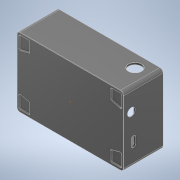
# Autodesk Inventor part: enclosure_bot
Saved by Autodesk Inventor 2021 (Build 250183000, 183)
## iProperties
Created: 2020-12-16
Part Number: enclosure_bot
Material: Generic
Document SubType Name: Modeling
Designer: oskar
Density: 1 g/cm^3
Appearance: Default
Author: oskar
## iProperties of the stored document _3DPrint.ipt
Created: 2020-12-16
Part Number: _3DPrint
Material: Generic
Document SubType Name: Modeling
Designer: oskar
Density: 1 g/cm^3
Appearance: Default
Author: oskar
Autodesk Inventor part; units mm, degrees
ref_plane "YZ Plane" through (0, 0, 0) normal (1, 0, 0) x (0, 1, 0)
ref_plane "XZ Plane" through (0, 0, 0) normal (0, 1, 0) x (-1, 0, 0)
ref_plane "XY Plane" through (0, 0, 0) normal (0, 0, 1) x (1, 0, 0)
ref_plane "Work Plane1" through (-0.485, 4.902, 9.06) normal (0, 0, 1) x (1, 0, 0)
sketch "Sketch1" plane through (-0.485, 4.902, 9.06) normal (0, 0, 1) x (1, 0, 0)
  line L0 (-52.815, 27.598) -> (47.185, 27.598)
  line L1 (47.185, 27.598) -> (47.185, -37.402)
  line L2 (47.185, -37.402) -> (-52.815, -37.402)
  line L3 (-52.815, -37.402) -> (-52.815, 27.598)
  line L4 (-52.815, 27.598) -> (47.185, -37.402) construction
  line L5 (47.185, 27.598) -> (-52.815, -37.402) construction
  line L6 (46.185, -13.982) -> (46.185, -20.322) projected
  line L7 (0.485, -4.902) -> (-19.0054, -4.902) construction
  point P0 (-2.815, -4.902)
  point P1 (-2.815, -4.902)
  dimension "d0" = 100
  dimension "d1" = 65
  dimension "d2" = 1
  constraints: 14 end point, 3 midpoint, 2 horizontal, 2 parallel, 1 perpendicular, 1 point on line
  measures "d0" distance of L0.start L0.end
  measures "d1" distance of L2.end L0.start
  measures "d2" distance between parallel lines of L6 L1
extrude "Extrusion1" add sketch "Sketch1" along normal blind 2
sketch "Sketch2" plane through (-0.485, 4.902, 11.06) normal (0, 0, 1) x (1, 0, 0)
  line L0 (36.185, 25.098) -> (44.185, 25.098)
  line L1 (45.185, 24.098) -> (45.185, 14.0681)
  line L2 (43.9425, 13.098) -> (35.9425, 15.098)
  line L3 (35.185, 16.0681) -> (35.185, 24.098)
  arc A0 (36.185, 25.098) -> (35.185, 24.098) centre (36.185, 24.098) ccw
  arc A1 (45.185, 24.098) -> (44.185, 25.098) centre (44.185, 24.098) ccw
  arc A2 (43.9425, 13.098) -> (45.185, 14.0681) centre (44.185, 14.0681) ccw
  arc A3 (35.185, 16.0681) -> (35.9425, 15.098) centre (36.185, 16.0681) ccw
  line L4 (-2.815, -4.902) -> (-2.815, 4.2729) construction
  line L5 (-2.815, -4.902) -> (-9.8185, -4.902) construction
  line L6 (-41.815, 25.098) -> (-49.815, 25.098)
  line L7 (-50.815, 24.098) -> (-50.815, 14.0681)
  line L8 (-49.5725, 13.098) -> (-41.5725, 15.098)
  line L9 (-40.815, 16.0681) -> (-40.815, 24.098)
  arc A4 (-40.815, 24.098) -> (-41.815, 25.098) centre (-41.815, 24.098) ccw
  arc A5 (-49.815, 25.098) -> (-50.815, 24.098) centre (-49.815, 24.098) ccw
  arc A6 (-50.815, 14.0681) -> (-49.5725, 13.098) centre (-49.815, 14.0681) ccw
  arc A7 (-41.5725, 15.098) -> (-40.815, 16.0681) centre (-41.815, 16.0681) ccw
  line L10 (36.185, -34.902) -> (44.185, -34.902)
  line L11 (45.185, -33.902) -> (45.185, -23.8721)
  line L12 (43.9425, -22.902) -> (35.9425, -24.902)
  line L13 (35.185, -25.8721) -> (35.185, -33.902)
  arc A8 (35.185, -33.902) -> (36.185, -34.902) centre (36.185, -33.902) ccw
  arc A9 (44.185, -34.902) -> (45.185, -33.902) centre (44.185, -33.902) ccw
  arc A10 (45.185, -23.8721) -> (43.9425, -22.902) centre (44.185, -23.8721) ccw
  arc A11 (35.9425, -24.902) -> (35.185, -25.8721) centre (36.185, -25.8721) ccw
  line L14 (-41.815, -34.902) -> (-49.815, -34.902)
  line L15 (-50.815, -33.902) -> (-50.815, -23.8721)
  line L16 (-49.5725, -22.902) -> (-41.5725, -24.902)
  line L17 (-40.815, -25.8721) -> (-40.815, -33.902)
  arc A12 (-41.815, -34.902) -> (-40.815, -33.902) centre (-41.815, -33.902) ccw
  arc A13 (-50.815, -33.902) -> (-49.815, -34.902) centre (-49.815, -33.902) ccw
  arc A14 (-49.5725, -22.902) -> (-50.815, -23.8721) centre (-49.815, -23.8721) ccw
  arc A15 (-40.815, -25.8721) -> (-41.5725, -24.902) centre (-41.815, -25.8721) ccw
  line L18 (47.185, -37.402) -> (47.185, 27.598) projected
  line L19 (-52.815, -37.402) -> (47.185, -37.402) projected
  point P0 (0.485, -4.902)
  dimension "d5" = 1
  dimension "d6" = 10
  dimension "d7" = 10
  dimension "d8" = 12
  dimension "d9" = 60
  dimension "d10" = 96
  dimension "d11" = 2
  dimension "d12" = 2.5
  constraints: 36 end point, 36 symmetric about line, 32 point on circle, 16 centre point, 8 tangent, 3 equal radius, 2 horizontal, 1 parallel, 1 perpendicular, 1 vertical, 12 other
  measures "d5" radius of A0
  measures "d6" distance between parallel lines of L3 L1
  measures "d7" distance from line of L2.end L0
  measures "d8" distance from line of L2.start L0
  measures "d9" distance between parallel lines of L0 L10
  measures "d10" distance between parallel lines of L7 L1
  measures "d11" distance between parallel lines of L18 L11
  measures "d12" distance between parallel lines of L19 L10
extrude "top" cut sketch "Sketch2" against normal blind 1.2
sketch "Sketch4" plane through (46.7, -32.5, 9.06) normal (1, 0, 0) x (0, 0, -1)
  line L0 (5.85, 17.08) -> (5.7, 17.08) construction
  line L1 (5.85, 17.08) -> (5.85, 23.42) construction
  line L2 (5.85, 23.42) -> (5.7, 23.42) construction
  line L3 (5.7, 23.42) -> (5.7, 17.08) construction
  arc A0 (5.7, 17.08) -> (7, 15.78) centre (7, 17.08) ccw construction
  line L4 (7, 15.93) -> (7, 15.78) construction
  arc A1 (5.85, 17.08) -> (7, 15.93) centre (7, 17.08) ccw construction
  line L5 (5.85, 17.08) -> (5.7, 17.08) construction
  line L6 (7.71, 15.93) -> (7.71, 15.78) construction
  line L7 (7.71, 15.93) -> (7, 15.93) construction
  line L8 (7, 15.93) -> (7, 15.78) construction
  line L9 (7, 15.78) -> (7.71, 15.78) construction
  arc A2 (7.71, 15.78) -> (9.01, 17.08) centre (7.71, 17.08) ccw construction
  line L10 (8.86, 17.08) -> (9.01, 17.08) construction
  arc A3 (7.71, 15.93) -> (8.86, 17.08) centre (7.71, 17.08) ccw construction
  line L11 (7.71, 15.93) -> (7.71, 15.78) construction
  line L12 (8.86, 20.6) -> (9.01, 20.6) construction
  line L13 (8.86, 20.6) -> (8.86, 17.08) construction
  line L14 (8.86, 17.08) -> (9.01, 17.08) construction
  line L15 (9.01, 17.08) -> (9.01, 20.6) construction
  arc A4 (7, 24.72) -> (5.7, 23.42) centre (7, 23.42) ccw construction
  line L16 (5.85, 23.42) -> (5.7, 23.42) construction
  arc A5 (7, 24.57) -> (5.85, 23.42) centre (7, 23.42) ccw construction
  line L17 (7, 24.57) -> (7, 24.72) construction
  line L18 (7, 24.57) -> (7, 24.72) construction
  line L19 (7, 24.57) -> (7.71, 24.57) construction
  line L20 (7.71, 24.57) -> (7.71, 24.72) construction
  line L21 (7.71, 24.72) -> (7, 24.72) construction
  arc A6 (9.01, 23.42) -> (7.71, 24.72) centre (7.71, 23.42) ccw construction
  line L22 (7.71, 24.57) -> (7.71, 24.72) construction
  arc A7 (8.86, 23.42) -> (7.71, 24.57) centre (7.71, 23.42) ccw construction
  line L23 (8.86, 23.42) -> (9.01, 23.42) construction
  line L24 (8.86, 23.42) -> (9.01, 23.42) construction
  line L25 (8.86, 23.42) -> (8.86, 20.65) construction
  line L26 (8.86, 20.65) -> (9.01, 20.65) construction
  line L27 (9.01, 20.65) -> (9.01, 23.42) construction
  line L28 (0, 0) -> (0, 65) projected
  line L29 (0, 0) -> (35, 0)
  line L30 (35, 0) -> (35, 65)
  line L31 (35, 65) -> (0, 65)
  line L32 (0, 65) -> (0, 0)
  circle A8 centre (5.3355, 45.2339) radius 1 construction
  circle A9 centre (5.3355, 45.2339) radius 3.5
  line L33 (7.71, 15.58) -> (7, 15.58)
  line L34 (5.5, 17.08) -> (5.5, 23.42)
  line L35 (7, 24.92) -> (7.71, 24.92)
  line L36 (9.21, 23.42) -> (9.21, 17.08)
  line L37 (9.21, 15.58) -> (5.5, 24.92) construction
  line L38 (5.5, 15.58) -> (9.21, 24.92) construction
  arc A10 (5.5, 17.08) -> (7, 15.58) centre (7, 17.08) ccw
  arc A11 (7.71, 15.58) -> (9.21, 17.08) centre (7.71, 17.08) ccw
  arc A12 (7, 24.92) -> (5.5, 23.42) centre (7, 23.42) ccw
  arc A13 (9.21, 23.42) -> (7.71, 24.92) centre (7.71, 23.42) ccw
  line L39 (1.66, 38.1339) -> (9.06, 38.1339)
  line L40 (9.06, 38.1339) -> (9.06, 49.1339)
  line L41 (9.06, 49.1339) -> (1.66, 49.1339)
  line L42 (1.66, 49.1339) -> (1.66, 38.1339)
  line L43 (1.66, 38.1339) -> (9.06, 49.1339) construction
  line L44 (9.06, 38.1339) -> (1.66, 49.1339) construction
  line L45 (8.0855, 38.9489) -> (2.0155, 38.9489) construction
  line L46 (2, 54.598) -> (5.6442, 54.5983) construction
  line L47 (2, 54.598) -> (2, 37.402) construction
  line L48 (9.06, 60) -> (9.06, 5) construction
  line L49 (5.6442, 37.4017) -> (2, 37.402) construction
  point P0 (9.06, 32.5)
  point P1 (7.355, 20.25)
  point P2 (5.36, 43.6339)
  dimension "d15" = 35
  dimension "d16" = 7
  dimension "d17" = 1.5
  dimension "d18" = 0.2
  dimension "d19" = 0.2
  dimension "d20" = 0.2
  dimension "d21" = 0.2
  dimension "d22" = 7.4
  dimension "d23" = 11
  dimension "d24" = 3.9
  constraints: 32 end point, 9 point on line, 8 point on circle, 8 tangent, 6 parallel, 5 centre point, 4 midpoint, 3 equal radius, 3 horizontal, 3 perpendicular, 1 coincident, 1 collinear
  measures "d15" distance of L30.end L31.end
  measures "d16" diameter of A9
  measures "d17" radius of A10
  measures "d18" distance between parallel lines of L21 L35
  measures "d19" distance between parallel lines of L33 L9
  measures "d20" distance between parallel lines of L15 L36
  measures "d21" distance between parallel lines of L34 L3
  measures "d22" distance between parallel lines of L42 L48
  measures "d23" distance between parallel lines of L39 L41
  measures "d24" distance from line of A8.centre L41
extrude "Extrusion3" add sketch "Sketch4" against normal blind 1.6 contours L28 L31 L30 L29
sketch "Sketch6" plane through (46.7, -32.5, 11.06) normal (1, 0, 0) x (0, 0, -1)
  line L0 (3.66, 38.1339) -> (3.66, 49.1339) projected
  line L1 (3.66, 49.1339) -> (11.06, 49.1339) projected
  line L2 (11.06, 49.1339) -> (11.06, 38.1339) projected
  line L3 (11.06, 38.1339) -> (3.66, 38.1339) projected
  line L4 (11.21, 23.42) -> (11.21, 17.08) projected
  arc A0 (9.71, 15.58) -> (11.21, 17.08) centre (9.71, 17.08) ccw projected
  line L5 (9.71, 15.58) -> (9, 15.58) projected
  arc A1 (7.5, 17.08) -> (9, 15.58) centre (9, 17.08) ccw projected
  line L6 (7.5, 17.08) -> (7.5, 23.42) projected
  arc A2 (9, 24.92) -> (7.5, 23.42) centre (9, 23.42) ccw projected
  line L7 (9, 24.92) -> (9.71, 24.92) projected
  arc A3 (11.21, 23.42) -> (9.71, 24.92) centre (9.71, 23.42) ccw projected
  line L8 (37, 65) -> (0, 65) projected
  line L9 (0, 0) -> (0, 65) projected
  line L10 (37, 0) -> (0, 0) projected
  line L11 (37, 0) -> (37, 65) projected
  circle A4 centre (7.3355, 45.2339) radius 1 projected
  circle A5 centre (7.3355, 45.2339) radius 3.5
  point P0 (11.06, 32.5)
  dimension "d27" = 7
  constraints: 1 centre point, 1 coincident
  measures "d27" diameter of A5
extrude "Extrusion4" add sketch "Sketch6" against normal blind 0.4 contours L0 L1 L2 L3
sketch "Sketch7" plane through (-53.3, 32.5, 11.06) normal (0, 1, 0) x (1, 0, 0)
  line L0 (98.4, 37) -> (98.4, 2) projected
  line L1 (98.4, 2) -> (0, 2)
  line L2 (0, 2) -> (0, 37)
  line L3 (0, 37) -> (98.4, 37)
  line L4 (98.4, 37) -> (98.4, 2)
  point P0 (53.3, 11.06)
  constraints: 8 end point, 2 parallel, 1 horizontal, 1 perpendicular
extrude "Extrusion5" add sketch "Sketch7" against normal blind 2
sketch "Sketch8" plane through (-53.3, -32.5, 11.06) normal (0, -1, 0) x (1, 0, 0)
  line L0 (0, -2) -> (98.4, -2)
  line L1 (98.4, -2) -> (98.4, -37)
  line L2 (98.4, -37) -> (0, -37)
  line L3 (0, -37) -> (0, -2)
  point P0 (53.3, -11.06)
  constraints: 8 end point, 2 coincident, 2 parallel, 1 horizontal, 1 perpendicular
extrude "Extrusion6" add sketch "Sketch8" against normal blind 2
sketch "Sketch9" plane through (-53.3, -32.5, 11.06) normal (-1, 0, 0) x (0, 0, 1)
  line L0 (-37, 63) -> (-2, 63)
  line L1 (-2, 63) -> (-2, 2)
  line L2 (-2, 2) -> (-37, 2)
  line L3 (-37, 2) -> (-37, 63)
  point P0 (-11.06, 32.5)
  constraints: 8 end point, 3 coincident, 2 parallel, 1 horizontal, 1 perpendicular
extrude "Extrusion7" add sketch "Sketch9" against normal blind 2
fillet "Fillet1" radius 3 8 edges at (-53.3, 32.5, -7.44) (-53.3, -32.5, -7.44) (46.7, 32.5, -7.44) (-51.3, 30.5, -8.44) (-51.3, -30.5, -8.44) (45.1, -30.5, -8.44) (46.7, -32.5, -7.44) (45.1, 30.5, -8.44)
fillet "Fillet2" radius 0.3 40 edges at (45.8213, 31.6213, 11.06) (-3.3, 32.5, 11.06) (-52.4213, 31.6213, 11.06) (-53.3, 0, 11.06) (-52.4213, -31.6213, 11.06) (-3.3, -32.5, 11.06) (45.8213, -31.6213, 11.06) (46.7, 0, 11.06) (34.9118, 20.3547, 11.06) (34.7, 24.9851, 11.06) (34.9929, 29.7071, 11.06) (39.7, 30, 11.06) (44.4071, 29.7071, 11.06) (44.7, 23.9851, 11.06) (44.3154, 18.1819, 11.06) (39.4575, 19, 11.06) (34.9118, -20.3547, 11.06) (39.4575, -19, 11.06) (44.3154, -18.1819, 11.06) (44.7, -23.9851, 11.06) (44.4071, -29.7071, 11.06) (39.7, -30, 11.06) (34.9929, -29.7071, 11.06) (34.7, -24.9851, 11.06) (-41.5929, -29.7071, 11.06) (-46.3, -30, 11.06) (-51.0071, -29.7071, 11.06) (-51.3, -23.9851, 11.06) (-50.9154, -18.1819, 11.06) (-46.0575, -19, 11.06) (-41.5118, -20.3547, 11.06) (-41.3, -24.9851, 11.06) (-50.9154, 18.1819, 11.06) (-51.3, 23.9851, 11.06) (-51.0071, 29.7071, 11.06) (-46.3, 30, 11.06) (-41.5929, 29.7071, 11.06) (-41.3, 24.9851, 11.06) (-41.5118, 20.3547, 11.06) (-46.0575, 19, 11.06)
sketch "Sketch10" plane through (-50.3, 32.5, -25.94) normal (0, 1, 0) x (1, 0, 0)
  circle A0 centre (82.4, -11.7) radius 6
  line L0 (92.4, -35) -> (92.4, 0) projected
  line L1 (94, -36.7) -> (0, -36.7) projected
  point P0 (50.3, -25.94)
  dimension "d39" = 12
  dimension "d40" = 10
  dimension "d41" = 25
  constraints: 1 centre point
  measures "d39" diameter of A0
  measures "d40" distance from line of A0.centre L0
  measures "d41" distance from line of L1 A0.centre
extrude "Extrusion8" cut sketch "Sketch10" against normal up to next
fillet "Fillet3" radius 0.2 24 edges at (45.1, -7.58, 1.705) (45.1, -8.0193, 3.1207) (45.1, -12.25, 3.56) (45.1, -16.4807, 3.1207) (45.1, -16.92, 1.705) (45.1, -16.4807, 0.2893) (45.1, -12.25, -0.15) (45.1, -8.0193, 0.2893) (46.7, -12.25, -0.15) (46.7, -16.4807, 0.2893) (46.7, -16.92, 1.705) (46.7, -16.4807, 3.1207) (46.7, -12.25, 3.56) (46.7, -8.0193, 3.1207) (46.7, -7.58, 1.705) (46.7, -8.0193, 0.2893) (46.7, 12.7339, 7.2245) (46.3, 12.7339, 7.2245) (45.1, 11.1339, 0) (45.1, 16.6339, 3.7) (45.1, 11.1339, 7.4) (45.1, 5.6339, 3.7) (26.1, 30.5, -14.24) (26.1, 32.5, -14.24)
sketch "Sketch11" plane through (46.7, -29.5, -25.94) normal (0, 0, -1) x (-1, 0, 0)
  arc A0 (0, 0) -> (3, -3) centre (3, 0) ccw projected
  line L0 (3, -3) -> (97, -3) projected
  arc A1 (97, -3) -> (100, 0) centre (97, 0) ccw projected
  line L1 (100, 59) -> (100, 0) projected
  arc A2 (100, 59) -> (97, 62) centre (97, 59) ccw projected
  line L2 (3, 62) -> (97, 62) projected
  arc A3 (3, 62) -> (0, 59) centre (3, 59) ccw projected
  line L3 (0, 0) -> (0, 59) projected
  arc A4 (1.6, 2) -> (4.6, -1) centre (4.6, 2) ccw projected
  line L4 (1.6, 57) -> (1.6, 2) projected
  arc A5 (4.6, 60) -> (1.6, 57) centre (4.6, 57) ccw projected
  line L5 (95, 60) -> (4.6, 60) projected
  arc A6 (98, 57) -> (95, 60) centre (95, 57) ccw projected
  line L6 (98, 2) -> (98, 57) projected
  arc A7 (95, -1) -> (98, 2) centre (95, 2) ccw projected
  line L7 (4.6, -1) -> (95, -1) projected
  point P0 (46.7, 29.5)
extrude "Extrusion9" add sketch "Sketch11" against normal blind 2 separate body contours L4 A5 L5 A6 L6 A7 L7 A4
sketch "Sketch12" plane through (46.7, -29.5, -25.94) normal (0, 0, -1) x (-1, 0, 0)
  arc A0 (0, 0) -> (3, -3) centre (3, 0) ccw projected
  line L0 (3, -3) -> (97, -3) projected
  arc A1 (97, -3) -> (100, 0) centre (97, 0) ccw projected
  line L1 (100, 59) -> (100, 0) projected
  arc A2 (100, 59) -> (97, 62) centre (97, 59) ccw projected
  line L2 (3, 62) -> (97, 62) projected
  arc A3 (3, 62) -> (0, 59) centre (3, 59) ccw projected
  line L3 (0, 0) -> (0, 59) projected
  arc A4 (1.6, 2) -> (4.6, -1) centre (4.6, 2) ccw projected
  line L4 (1.6, 57) -> (1.6, 2) projected
  arc A5 (4.6, 60) -> (1.6, 57) centre (4.6, 57) ccw projected
  line L5 (95, 60) -> (4.6, 60) projected
  arc A6 (98, 57) -> (95, 60) centre (95, 57) ccw projected
  line L6 (98, 2) -> (98, 57) projected
  arc A7 (95, -1) -> (98, 2) centre (95, 2) ccw projected
  line L7 (4.6, -1) -> (95, -1) projected
  point P0 (46.7, 29.5)
extrude "Extrusion10" add sketch "Sketch12" along normal blind 2 contours L3 A3 L2 A2 L1 A1 L0 A0 | L4 A5 L5 A6 L6 A7 L7 A4 bodies 2
thicken "Thicken1" operation add thickness 0.1 both sides no extend neighbours yes toward (0, -1, 0) bodies 2 faces at (-18.1667, 30.5, -25.2733) (42.3242, 30.4916, -25.2733) (45.1, 9.1667, -25.2733) (-48.5242, 30.4916, -24.6067) (-51.3, -9.1667, -25.2733) (-48.5242, -30.4916, -25.2733) (11.9667, -30.5, -25.2733) (43.6, -30.0981, -24.6067)
ref_plane "Work Plane2" through (-41.2, -27.5, -25.94) normal (-1, 0, 0) x (0, 0, 1)
sketch "Sketch14" plane through (-41.2, -27.5, -25.94) normal (-1, 0, 0) x (0, 0, 1)
  arc A0 (6, 53.1102) -> (2.2, 43.5695) centre (12.072, 45.1646) ccw
  line L0 (-46.8982, 30.6102) -> (-15.0993, 30.6102) construction
  arc A1 (2.2, 17.6509) -> (6, 8.1102) centre (12.072, 16.0557) ccw
  arc A2 (2.2, 17.6509) -> (2.2, 43.5695) centre (-78, 30.6102) ccw
  line L1 (6, 53.1102) -> (2, 53.1102)
  line L2 (2, 53.1102) -> (2, 8.1102)
  line L3 (2, 8.1102) -> (6, 8.1102)
  line L4 (2, 55) -> (2, 0) projected
  point P0 (25.94, 27.5)
  dimension "d51" = 10
  dimension "d52" = 45
  dimension "d53" = 0.2
  dimension "d54" = 4
  dimension "d55" = 80
  constraints: 8 end point, 6 point on circle, 3 centre point, 3 horizontal, 3 symmetric about line, 1 collinear, 1 perpendicular, 1 tangent, 1 other
  measures "d51" radius of A0
  measures "d52" distance between parallel lines of L1 L3
  measures "d53" distance from line of L2 A0.end
  measures "d54" distance from line of L2 L1.start
  measures "d55" distance from line of L2 A2.centre
extrude "Extrusion11" add sketch "Sketch14" against normal blind 60 bodies 2
sketch "Sketch15" plane through (-0.485, 4.902, 9.06) normal (0, 0, -1) x (-1, 0, 0)
  circle A0 centre (-0.485, -4.1052) radius 2.5
  point P0 (-0.485, -4.902)
  dimension "d58" = 5
  constraints: 1 centre point
  measures "d58" diameter of A0
extrude "Extrusion12" cut sketch "Sketch15" against normal blind 1 bodies 1
equation "\"d3\" = t_wall"
equation "\"d18\" = d20"
equation "\"d19\" = d20"
equation "\"d21\" = d20"
equation "\"d30\" = t_wall"
equation "\"d32\" = t_wall"
equation "\"d34\" = t_wall"
equation "\"d42\" = t_wall"
equation "\"d44\" = t_wall"
equation "\"d46\" = t_wall"
equation "\"d59\" = 0.5 * t_wall"
equation "\"t_wall\" = 2"
body "Solid1"
body "Solid2"
